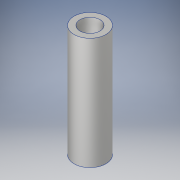
# Autodesk Inventor part: spacer x
Saved by Autodesk Inventor 2019 (Build 230136000, 136)
## iProperties
Created: 2018-08-04
Part Number: spacer x
Material: Aluminum 6061
Document SubType Name: Modeling
Designer: torba
Density: 2.7 g/cm^3
Appearance: Aluminum - Flat
Author: torba
Autodesk Inventor part; units mm, degrees
ref_plane "YZ Plane" through (0, 0, 0) normal (1, 0, 0) x (0, 1, 0)
ref_plane "XZ Plane" through (0, 0, 0) normal (0, 1, 0) x (-1, 0, 0)
ref_plane "XY Plane" through (0, 0, 0) normal (0, 0, 1) x (1, 0, 0)
sketch "Sketch1" plane through (0, 0, 0) normal (0, 1, 0) x (-1, 0, 0)
  circle A0 centre (0, 0) radius 4
  circle A1 centre (0, 0) radius 2.5
  dimension "d2" = 5
  dimension "d3" = 8
  constraints: 2 centre point, 2 coincident
  measures "d2" diameter of A1
  measures "d3" diameter of A0
extrude "Extrusion1" add sketch "Sketch1" along normal blind 28.15
body "Solid1"
